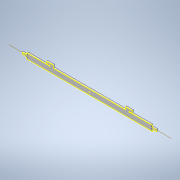
# Autodesk Inventor part: rod_2
Saved by Autodesk Inventor 2022 (Build 260153000, 153)
## iProperties
Created: 2023-04-07
Part Number: rod_2
Material: 一般
Document SubType Name: Modeling
Designer: may9c
Density: 1 g/cm^3
Appearance: 預設
Author: may9c
Autodesk Inventor part; units mm, degrees
ref_plane "YZ Plane" through (0, 0, 0) normal (1, 0, 0) x (0, 1, 0)
ref_plane "XY Plane" through (0, 0, 0) normal (0, 0, 1) x (1, 0, 0)
sketch "草圖1" plane through (0, 0, 0) normal (0, 0, 1) x (1, 0, 0)
  line L0 (0, 6) -> (0, -6)
  line L1 (0, -6) -> (-144, -6)
  line L2 (-144, -6) -> (-144, 6)
  line L3 (-153, 2) -> (-144, 2)
  line L4 (-144, 2) -> (-144, -2)
  line L5 (-144, -2) -> (-153, -2)
  line L6 (-153, -2) -> (-153, 2)
  line L7 (-214.2, 0) -> (214.2, 0) projected
  line L8 (0, -9.6) -> (0, 15.6) projected
  line L9 (0, -6) -> (144, -6)
  line L10 (144, -6) -> (144, 6)
  line L11 (153, 2) -> (144, 2)
  line L12 (144, -2) -> (153, -2)
  line L13 (153, -2) -> (153, 2)
  line L14 (-153, -2) -> (-144, -2)
  line L15 (-144, -2) -> (-144, -6)
  line L16 (144, -6) -> (144, -2)
  line L17 (144, -2) -> (153, -2)
  line L18 (153, -2) -> (153, 2)
  line L19 (153, 2) -> (144, 2)
  line L20 (144, 2) -> (144, 6)
  line L21 (-144, 6) -> (-144, 2)
  line L22 (-144, 2) -> (-153, 2)
  line L23 (-153, 2) -> (-153, -2)
  line L24 (-97.5, 7) -> (-97.5, 12)
  line L25 (-97.5, 12) -> (-82.5, 12)
  line L26 (-90, 7) -> (-97.5, 7)
  line L27 (-82.5, 12) -> (-82.5, 6)
  line L28 (-90, 7) -> (-90, 5)
  line L29 (-90, 5) -> (-91, 5)
  line L30 (-91, 5) -> (-91, 6)
  line L31 (90, 7) -> (97.5, 7)
  line L32 (97.5, 7) -> (97.5, 12)
  line L33 (97.5, 12) -> (82.5, 12)
  line L34 (82.5, 12) -> (82.5, 6)
  line L35 (90, 7) -> (90, 5)
  line L36 (90, 5) -> (91, 5)
  line L37 (91, 5) -> (91, 6)
  line L38 (-144, 6) -> (-91, 6)
  line L39 (-82.5, 6) -> (82.5, 6)
  line L40 (91, 6) -> (144, 6)
  line L41 (-144, 6) -> (-91, 6)
  line L42 (-82.5, 6) -> (0, 6)
  line L43 (144, 6) -> (91, 6)
  line L44 (82.5, 6) -> (0, 6)
  point P0 (0, 0)
  dimension "d0" = 9
  dimension "d1" = 144
  dimension "d2" = 4
  constraints: 86 end point, 6 symmetric about line, 5 parallel, 3 horizontal, 3 perpendicular, 2 point on line, 1 collinear, 1 other
  measures "d0" distance between parallel lines of L6 L2
  measures "d1" distance of L2.end L0.start
  measures "d2" distance between parallel lines of L5 L3
extrude "擠出1" add sketch "草圖1" along normal blind 3
sketch "草圖2" plane through (0, 0, 3) normal (0, 0, 1) x (1, 0, 0)
  line L0 (-153, -2) -> (-144, -2) projected
  line L1 (-144, -2) -> (-144, -6) projected
  line L2 (-144, -6) -> (144, -6) projected
  line L3 (144, -6) -> (144, -2) projected
  line L4 (144, -2) -> (153, -2) projected
  line L5 (153, -2) -> (153, 2) projected
  line L6 (153, 2) -> (144, 2) projected
  line L7 (144, 2) -> (144, 6) projected
  line L8 (-91, 6) -> (-144, 6) projected
  line L9 (-144, 6) -> (-144, 2) projected
  line L10 (-144, 2) -> (-153, 2) projected
  line L11 (-153, 2) -> (-153, -2) projected
  line L12 (144, 6) -> (91, 6) projected
  line L13 (91, 6) -> (91, 5) projected
  line L14 (91, 5) -> (90, 5) projected
  line L15 (90, 5) -> (90, 7) projected
  line L16 (90, 7) -> (97.5, 7) projected
  line L17 (97.5, 7) -> (97.5, 12) projected
  line L18 (97.5, 12) -> (82.5, 12) projected
  line L19 (82.5, 12) -> (82.5, 6) projected
  line L20 (82.5, 6) -> (-82.5, 6) projected
  line L21 (-82.5, 6) -> (-82.5, 12) projected
  line L22 (-82.5, 12) -> (-97.5, 12) projected
  line L23 (-97.5, 12) -> (-97.5, 7) projected
  line L24 (-97.5, 7) -> (-90, 7) projected
  line L25 (-90, 7) -> (-90, 5) projected
  line L26 (-90, 5) -> (-91, 5) projected
  line L27 (-91, 5) -> (-91, 6) projected
  point P0 (0, 0)
ref_plane "工作平面1" through (0, 0, 1.5) normal (0, 0, 1) x (1, 0, 0)
move faces "移動1" translate (-3, 0, 0) faces at (144, 3.3333, 1) (144, -4.6667, 1)
move faces "移動2" translate (3, 0, 0) faces at (-144, 4.6667, 1) (-144, -3.3333, 1)
